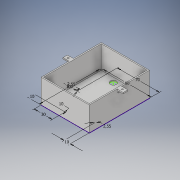
# Autodesk Inventor part: Contenedor Puente H v1.0
Saved by Autodesk Inventor 2019 (Build 230136000, 136)
## iProperties
Created: 2018-07-22
Part Number: Contenedor Puente H v1.0
Material: Genérico
Document SubType Name: Modeling
Designer: Francisco
Density: 1 g/cm^3
Appearance: Valor por defecto
Author: Francisco
## iProperties of the stored document Contenedor Puente H v1_3DPrint.ipt
Created: 2018-07-22
Part Number: Contenedor Puente H v1_3DPrint
Material: Genérico
Document SubType Name: Modeling
Designer: Francisco
Density: 1 g/cm^3
Appearance: Valor por defecto
Author: Francisco
Autodesk Inventor part; units mm, degrees
ref_plane "YZ Plane" through (0, 0, 0) normal (1, 0, 0) x (0, 1, 0)
ref_plane "XZ Plane" through (0, 0, 0) normal (0, 1, 0) x (-1, 0, 0)
ref_plane "XY Plane" through (0, 0, 0) normal (0, 0, 1) x (1, 0, 0)
sketch "Base" plane through (0, 0, 0) normal (0, 1, 0) x (-1, 0, 0)
  line L0 (-40, 50) -> (40, 50)
  line L1 (40, 50) -> (40, -50)
  line L2 (40, -50) -> (-40, -50)
  line L3 (-40, -50) -> (-40, 50)
  line L4 (-40, 50) -> (40, -50) construction
  line L5 (40, 50) -> (-40, -50) construction
  circle A0 centre (10, 40) radius 5
  circle A1 centre (-10, 40) radius 5
  circle A2 centre (10, -40) radius 5
  circle A3 centre (-10, -40) radius 5
  circle A4 centre (-30, 30) radius 1.275
  circle A5 centre (-30, -30) radius 1.275
  circle A6 centre (30, 0) radius 1.275
  line L6 (38, -48) -> (38, 48)
  line L7 (38, 48) -> (-38, 48)
  line L8 (-38, 48) -> (-38, -48)
  line L9 (-38, -48) -> (38, -48)
  point P0 (0, 0)
  dimension "d0" = 80
  dimension "d1" = 100
  dimension "d2" = 30
  dimension "d3" = 10
  dimension "d4" = 10
  dimension "d6" = 10
  dimension "d7" = 2.55
  dimension "d8" = 70
  dimension "d10" = 2.55
  dimension "d11" = 2
  constraints: 20 end point, 7 centre point, 4 parallel, 3 coincident, 2 midpoint, 2 perpendicular, 1 horizontal, 3 other
  measures "d0" distance of L1.end L2.end
  measures "d1" distance of L0.end L1.end
  measures "d2" distance from line of point (10, 40) L1
  measures "d3" distance from line of L0 point (10, 40)
  measures "d4" diameter of A0
  measures "d6" distance from line of L3 point (-30, 30)
  measures "d7" diameter of A4
  measures "d8" distance from line of L3 point (30, 0)
  measures "d10" diameter of A6
  measures "d11" distance between parallel lines of L1 L6
extrude "Extrusión base" add sketch "Base" along normal blind 2 contours L9 L8 L7 L6
extrude "Paredes" add sketch "Base" along normal blind 40 contours L0 L1 L2 L3
sketch "Boceto2" plane through (-40, 0, -50) normal (-1, 0, 0) x (0, 0, 1)
  line L0 (0, 40) -> (100, 40) projected
  line L1 (98, 40) -> (2, 40) projected
  line L2 (46.25, 35) -> (53.75, 35)
  line L3 (53.75, 35) -> (53.75, 40)
  line L4 (53.75, 40) -> (46.25, 40)
  line L5 (46.25, 40) -> (46.25, 35)
  line L6 (46.25, 35) -> (53.75, 40) construction
  line L7 (53.75, 35) -> (46.25, 40) construction
  point P0 (50, 0)
  point P1 (50, 37.5)
  dimension "d16" = 2.5
  dimension "d17" = 7.5
  constraints: 12 end point, 2 midpoint, 2 parallel, 1 horizontal, 1 perpendicular, 1 point on line
  measures "d16" distance from line of L0 point (50, 37.5)
  measures "d17" distance of L4.end L3.end
extrude "Extrusión3" add sketch "Boceto2" along normal blind 2
mirror "Simetría1" about plane through (0, 0, 0) normal (1, 0, 0) of "Extrusión3"
sketch "Boceto3" plane through (-42, 0, -50) normal (-1, 0, 0) x (0, 0, 1)
  line L0 (53.75, 40) -> (46.25, 40) projected
  line L1 (53.75, 40) -> (53.75, 35) projected
  line L2 (46.25, 38) -> (53.75, 38)
  line L3 (53.75, 38) -> (53.75, 40)
  line L4 (53.75, 40) -> (46.25, 40)
  line L5 (46.25, 40) -> (46.25, 38)
  line L6 (46.25, 38) -> (53.75, 40) construction
  line L7 (53.75, 38) -> (46.25, 40) construction
  point P0 (50, 0)
  point P1 (50, 39)
  dimension "d20" = 1
  constraints: 12 end point, 2 midpoint, 2 parallel, 1 horizontal, 1 perpendicular
  measures "d20" distance from line of L0 point (50, 39)
extrude "Extrusión4" add sketch "Boceto3" along normal blind 8
mirror "Simetría2" about plane through (0, 0, 0) normal (1, 0, 0) of "Extrusión4"
sketch "Boceto4" plane through (0, 40, 0) normal (0, 1, 0) x (1, 0, 0)
  line L0 (-50, -3.75) -> (-50, 3.75) projected
  line L1 (-40, -3.75) -> (-50, -3.75) projected
  circle A0 centre (-45, 0) radius 1.275
  point P0 (0, 0)
  dimension "d23" = 5
  dimension "d24" = 3.75
  dimension "d25" = 2.55
  constraints: 1 centre point, 1 coincident
  measures "d23" distance from line of L0 point (-45, 0)
  measures "d24" distance from line of L1 point (-45, 0)
  measures "d25" diameter of A0
hole "Agujero1" at (-45, 40, 0) direction (0, -1, 0) diameter 2.55 end through all
mirror "Simetría3" about plane through (0, 0, 0) normal (1, 0, 0) of "Agujero1"
